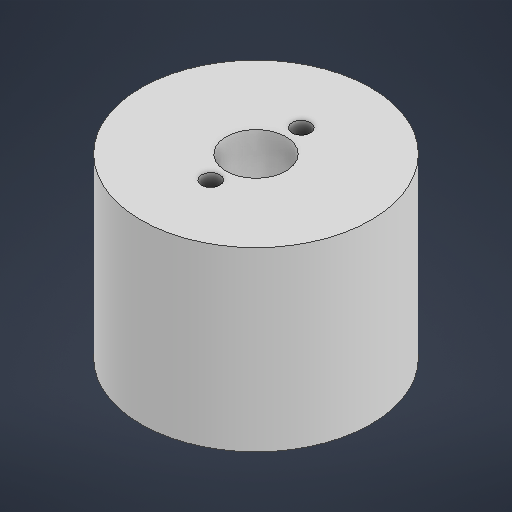
# Autodesk Inventor part: PolarisPost_HeightAdjustment_0p5in_Machined
Saved by Autodesk Inventor 2026 (Build 300175000, 175)
## iProperties
Created: 2024-01-08
Part Number: PolarisPost_HeightAdjustment_0p5in_Machined
Material: Generic
Document SubType Name: Modeling
Designer: monolithic
Density: 1 g/cm^3
Appearance: Default
Author: monolithic
Autodesk Inventor part; units mm, degrees
ref_plane "YZ Plane" through (0, 0, 0) normal (1, 0, 0) x (0, 1, 0)
ref_plane "XZ Plane" through (0, 0, 0) normal (0, 1, 0) x (-1, 0, 0)
ref_plane "XY Plane" through (0, 0, 0) normal (0, 0, 1) x (1, 0, 0)
sketch "Sketch1" plane through (0, 0, 0) normal (0, 1, 0) x (-1, 0, 0)
  circle A0 centre (0, 0) radius 12.7
  circle A1 centre (0, 0) radius 3.302
  dimension "d0" = 25.4
  dimension "d1" = 6.604
  constraints: 2 centre point, 2 coincident
  measures "d0" diameter of A0
  measures "d1" diameter of A1
extrude "Extrusion1" add sketch "Sketch1" along normal blind 19.558
sketch "Sketch2" plane through (0, 19.558, 0) normal (0, 1, 0) x (1, 0, 0)
  line L0 (0, 0) -> (0, -5.004)
  line L1 (0, -5.004) -> (0, 0)
  line L2 (0, 0) -> (0, 5.004)
  circle A0 centre (0, -5.004) radius 1.0125
  circle A1 centre (0, 5.004) radius 1.0125
  dimension "d4" = 5.004
  dimension "d5" = 5.004
  dimension "d6" = 2.025
  dimension "d7" = 2.025
  constraints: 6 end point, 2 centre point, 2 coincident, 1 collinear, 1 point on line, 1 vertical
  measures "d4" distance of L0.start L0.end
  measures "d5" distance of L0.start L2.end
  measures "d6" diameter of A0
  measures "d7" diameter of A1
extrude "Extrusion2" cut sketch "Sketch2" against normal blind 4.445
sketch "Sketch3" plane through (0, 0, 0) normal (0, -1, 0) x (1, 0, 0)
  line L0 (0, 0) -> (0, 5.004)
  line L1 (0, 5.004) -> (0, -5.08)
  circle A0 centre (0, 5.004) radius 1.0125
  line L2 (0, 0) -> (0, -5.004)
  circle A1 centre (0, -5.08) radius 1.0125
  dimension "d10" = 5.004
  dimension "d15" = 2.025
  dimension "d16" = 5.004
  dimension "d17" = 2.025
  constraints: 6 end point, 2 centre point, 2 coincident, 2 point on line, 1 vertical
  measures "d10" distance of L0.start L0.end
  measures "d15" diameter of A0
  measures "d16" distance of L0.start L2.end
  measures "d17" diameter of A1
extrude "Extrusion3" cut sketch "Sketch3" against normal blind 4.445
body "Solid1"
